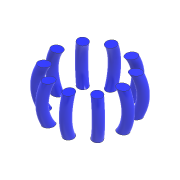
# Autodesk Inventor part: Roller_Gear
Saved by Autodesk Inventor 2022 (Build 260153000, 153)
## iProperties
Created: 2023-10-11
Part Number: Roller_Gear
Material: 一般
Document SubType Name: Modeling
Designer: JOU
Density: 1 g/cm^3
Appearance: 預設
Author: JOU
Autodesk Inventor part; units mm, degrees
ref_plane "YZ Plane" through (0, 0, 0) normal (1, 0, 0) x (0, 1, 0)
ref_plane "XY Plane" through (0, 0, 0) normal (0, 0, 1) x (1, 0, 0)
sketch "草圖1" plane through (0, 0, 0) normal (0, 0, 1) x (1, 0, 0)
  circle A0 centre (0, 0) radius 40
  dimension "d0" = 80
  constraints: 1 centre point, 1 coincident
  measures "d0" diameter of A0
sketch "草圖2" plane through (0, 0, 0) normal (0, 1, 0) x (-1, 0, 0)
  line L0 (40, 0) -> (-40, 0) projected
  circle A0 centre (40, 0) radius 5
  point P0 (0, 0)
  dimension "d1" = 10
  constraints: 1 centre point, 1 coincident
  measures "d1" diameter of A0
sketch "草圖2 outline for 掃掠1" plane through (0, 0, 0) normal (0, 1, 0) x (-1, 0, 0)
  circle A0 centre (40, 0) radius 5
sweep "掃掠1" add profiles "草圖2 outline for 掃掠1" path "草圖1"
pattern_circular "環形陣列1" count 5 over 360 about axis through (0, -10, 0) along (0, 1, 0)
ref_plane "工作平面1" through (0, 20, 0) normal (0, 1, 0) x (-1, 0, 0)
sketch "草圖5" plane through (0, 20, 0) normal (0, 1, 0) x (-1, 0, 0)
  circle A0 centre (0, 0) radius 45
  dimension "d8" = 90
  constraints: 1 centre point, 1 coincident
  measures "d8" diameter of A0
sketch "草圖5 outline for 擠出1" plane through (0, 20, 0) normal (0, 1, 0) x (-1, 0, 0)
  circle A0 centre (0, 0) radius 45
extrude "擠出1" cut sketch "草圖5 outline for 擠出1" along normal through all
mirror "鏡射1" about plane through (0, 0, 0) normal (0, 1, 0) of "擠出1"
